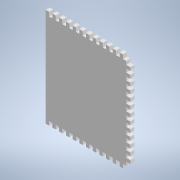
# Autodesk Inventor part: unlong
Saved by Autodesk Inventor 2022 (Build 260153000, 153)
## iProperties
Created: 2023-05-26
Part Number: unlong
Material: Типовые
Document SubType Name: Modeling
Designer: korsh624
Density: 1 g/cm^3
Appearance: По умолчанию
Author: korsh624
Autodesk Inventor part; units mm, degrees
ref_plane "YZ Plane" through (0, 0, 0) normal (1, 0, 0) x (0, 1, 0)
ref_plane "XZ Plane" through (0, 0, 0) normal (0, 1, 0) x (-1, 0, 0)
ref_plane "XY Plane" through (0, 0, 0) normal (0, 0, 1) x (1, 0, 0)
sketch "Эскиз1" plane through (0, 0, 0) normal (0, 0, 1) x (1, 0, 0)
  line L0 (0, 0) -> (5, 0) projected
  line L1 (5, 0) -> (5, 6) projected
  line L2 (0, 6) -> (5, 6) projected
  line L3 (0, 0) -> (0, 6) projected
  line L4 (10, 0) -> (15, 0) projected
  line L5 (15, 0) -> (15, 6) projected
  line L6 (10, 6) -> (15, 6) projected
  line L7 (10, 0) -> (10, 6) projected
  line L8 (20, 0) -> (25, 0) projected
  line L9 (25, 0) -> (25, 6) projected
  line L10 (20, 6) -> (25, 6) projected
  line L11 (20, 0) -> (20, 6) projected
  line L12 (30, 0) -> (35, 0) projected
  line L13 (35, 0) -> (35, 6) projected
  line L14 (30, 6) -> (35, 6) projected
  line L15 (30, 0) -> (30, 6) projected
  line L16 (40, 0) -> (45, 0) projected
  line L17 (45, 0) -> (45, 6) projected
  line L18 (40, 6) -> (45, 6) projected
  line L19 (40, 0) -> (40, 6) projected
  line L20 (50, 0) -> (55, 0) projected
  line L21 (55, 0) -> (55, 6) projected
  line L22 (50, 6) -> (55, 6) projected
  line L23 (50, 0) -> (50, 6) projected
  line L24 (60, 0) -> (65, 0) projected
  line L25 (65, 0) -> (65, 6) projected
  line L26 (60, 6) -> (65, 6) projected
  line L27 (60, 0) -> (60, 6) projected
  line L28 (70, 0) -> (75, 0) projected
  line L29 (75, 0) -> (75, 6) projected
  line L30 (70, 6) -> (75, 6) projected
  line L31 (70, 0) -> (70, 6) projected
  line L32 (80, 0) -> (85, 0) projected
  line L33 (85, 0) -> (85, 6) projected
  line L34 (80, 6) -> (85, 6) projected
  line L35 (80, 0) -> (80, 6) projected
  line L36 (90, 0) -> (95, 0) projected
  line L37 (95, 0) -> (95, 6) projected
  line L38 (90, 6) -> (95, 6) projected
  line L39 (90, 0) -> (90, 6) projected
  line L40 (100, 0) -> (105, 0) projected
  line L41 (105, 0) -> (105, 6) projected
  line L42 (100, 6) -> (105, 6) projected
  line L43 (100, 0) -> (100, 6) projected
  line L44 (110, 0) -> (115, 0) projected
  line L45 (115, 0) -> (115, 6) projected
  line L46 (110, 6) -> (115, 6) projected
  line L47 (110, 0) -> (110, 6) projected
  line L48 (115, 6) -> (120, 6) projected
  line L49 (120, 11) -> (120, 6) projected
  line L50 (120, 16) -> (120, 11) projected
  line L51 (120, 11) -> (126, 11) projected
  line L52 (126, 16) -> (126, 11) projected
  line L53 (120, 16) -> (126, 16) projected
  line L54 (0, 141) -> (5, 141) projected
  line L55 (5, 141) -> (5, 147) projected
  line L56 (0, 147) -> (5, 147) projected
  line L57 (0, 141) -> (0, 147) projected
  line L58 (15, 141) -> (15, 147) projected
  line L59 (10, 141) -> (15, 141) projected
  line L60 (15, 141) -> (15, 147) projected
  line L61 (10, 147) -> (15, 147) projected
  line L62 (10, 141) -> (10, 147) projected
  line L63 (20, 141) -> (25, 141) projected
  line L64 (25, 141) -> (25, 147) projected
  line L65 (20, 147) -> (25, 147) projected
  line L66 (20, 141) -> (20, 147) projected
  line L67 (30, 141) -> (35, 141) projected
  line L68 (35, 141) -> (35, 147) projected
  line L69 (30, 147) -> (35, 147) projected
  line L70 (30, 141) -> (30, 147) projected
  line L71 (40, 141) -> (45, 141) projected
  line L72 (45, 141) -> (45, 147) projected
  line L73 (40, 147) -> (45, 147) projected
  line L74 (40, 141) -> (40, 147) projected
  line L75 (50, 141) -> (55, 141) projected
  line L76 (55, 141) -> (55, 147) projected
  line L77 (50, 147) -> (55, 147) projected
  line L78 (50, 141) -> (50, 147) projected
  line L79 (60, 141) -> (65, 141) projected
  line L80 (65, 141) -> (65, 147) projected
  line L81 (60, 147) -> (65, 147) projected
  line L82 (60, 141) -> (60, 147) projected
  line L83 (70, 141) -> (75, 141) projected
  line L84 (75, 141) -> (75, 147) projected
  line L85 (70, 147) -> (75, 147) projected
  line L86 (70, 141) -> (70, 147) projected
  line L87 (80, 141) -> (85, 141) projected
  line L88 (85, 141) -> (85, 147) projected
  line L89 (80, 147) -> (85, 147) projected
  line L90 (80, 141) -> (80, 147) projected
  line L91 (90, 141) -> (95, 141) projected
  line L92 (95, 141) -> (95, 147) projected
  line L93 (90, 147) -> (95, 147) projected
  line L94 (90, 141) -> (90, 147) projected
  line L95 (100, 141) -> (105, 141) projected
  line L96 (105, 141) -> (105, 147) projected
  line L97 (100, 147) -> (105, 147) projected
  line L98 (100, 141) -> (100, 147) projected
  line L99 (110, 141) -> (115, 141) projected
  line L100 (115, 141) -> (115, 147) projected
  line L101 (110, 147) -> (115, 147) projected
  line L102 (110, 141) -> (110, 147) projected
  line L103 (115, 141) -> (120, 141) projected
  line L104 (120, 141) -> (120, 136) projected
  line L105 (120, 136) -> (120, 131) projected
  line L106 (120, 131) -> (126, 131) projected
  line L107 (126, 136) -> (126, 131) projected
  line L108 (120, 136) -> (126, 136) projected
  line L109 (120, 126) -> (120, 121) projected
  line L110 (120, 121) -> (126, 121) projected
  line L111 (126, 126) -> (126, 121) projected
  line L112 (120, 126) -> (126, 126) projected
  line L113 (120, 116) -> (120, 111) projected
  line L114 (120, 111) -> (126, 111) projected
  line L115 (126, 116) -> (126, 111) projected
  line L116 (120, 116) -> (126, 116) projected
  line L117 (120, 106) -> (120, 101) projected
  line L118 (120, 101) -> (126, 101) projected
  line L119 (126, 106) -> (126, 101) projected
  line L120 (120, 106) -> (126, 106) projected
  line L121 (120, 96) -> (120, 91) projected
  line L122 (120, 91) -> (126, 91) projected
  line L123 (126, 96) -> (126, 91) projected
  line L124 (120, 96) -> (126, 96) projected
  line L125 (120, 86) -> (120, 81) projected
  line L126 (120, 81) -> (126, 81) projected
  line L127 (126, 86) -> (126, 81) projected
  line L128 (120, 86) -> (126, 86) projected
  line L129 (120, 76) -> (120, 71) projected
  line L130 (120, 71) -> (126, 71) projected
  line L131 (126, 76) -> (126, 71) projected
  line L132 (120, 76) -> (126, 76) projected
  line L133 (120, 66) -> (120, 61) projected
  line L134 (120, 61) -> (126, 61) projected
  line L135 (126, 66) -> (126, 61) projected
  line L136 (120, 66) -> (126, 66) projected
  line L137 (120, 56) -> (120, 51) projected
  line L138 (120, 51) -> (126, 51) projected
  line L139 (126, 56) -> (126, 51) projected
  line L140 (120, 56) -> (126, 56) projected
  line L141 (120, 46) -> (120, 41) projected
  line L142 (120, 41) -> (126, 41) projected
  line L143 (126, 46) -> (126, 41) projected
  line L144 (120, 46) -> (126, 46) projected
  line L145 (120, 36) -> (120, 31) projected
  line L146 (120, 31) -> (126, 31) projected
  line L147 (126, 36) -> (126, 31) projected
  line L148 (120, 36) -> (126, 36) projected
  line L149 (120, 26) -> (120, 21) projected
  line L150 (120, 21) -> (126, 21) projected
  line L151 (126, 26) -> (126, 21) projected
  line L152 (120, 26) -> (126, 26) projected
  line L153 (0, 6) -> (120, 6)
  line L154 (120, 6) -> (120, 141)
  line L155 (120, 141) -> (0, 141)
  line L156 (0, 141) -> (0, 6)
  constraints: 2 end point, 1 vertical, 9 other
extrude "Выдавливание1" add sketch "Эскиз1" along normal blind 6
